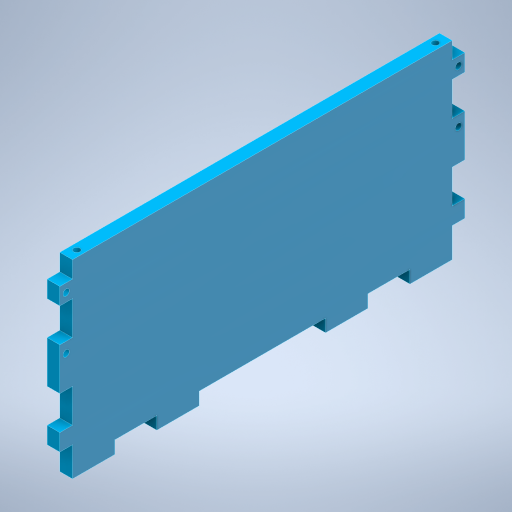
# Autodesk Inventor part: передняя стенка
Saved by Autodesk Inventor 2024.2 (Build 282272000, 272)
## iProperties
Created: 2025-11-20
Part Number: передняя стенка
Material: Типовые
Document SubType Name: Modeling
Designer: Zakhar
Density: 1 g/cm^3
Appearance: Небесно-голубой — нейтральный
Mass: 95.616 g
Surface Area: 351.84 cm^2
Volume: 95.616 cm^3
Author: Zakhar
Autodesk Inventor part; units mm, degrees
ref_plane "YZ Plane" through (0, 0, 0) normal (1, 0, 0) x (0, 1, 0)
ref_plane "XZ Plane" through (0, 0, 0) normal (0, 1, 0) x (-1, 0, 0)
ref_plane "XY Plane" through (0, 0, 0) normal (0, 0, 1) x (1, 0, 0)
sketch "Эскиз1" plane through (0, 0, 0) normal (1, 0, 0) x (0, 1, 0)
  line L0 (84, 90) -> (0, 90)
  line L1 (0, 90) -> (0, -90)
  line L2 (0, -90) -> (84, -90)
  line L3 (84, -90) -> (84, 90)
  line L4 (76, 90) -> (8, 90)
  line L5 (8, 90) -> (8, 96)
  line L6 (8, 96) -> (76, 96)
  line L7 (76, 96) -> (76, 90)
  line L8 (76, -90) -> (8, -90)
  line L9 (8, -90) -> (8, -96)
  line L10 (8, -96) -> (76, -96)
  line L11 (76, -96) -> (76, -90)
  line L12 (16, -96) -> (16, -90)
  line L13 (32, -96) -> (32, -90)
  line L14 (68, -96) -> (68, -90)
  line L15 (52, -96) -> (52, -90)
  line L16 (16, 90) -> (16, 96)
  line L17 (32, 90) -> (32, 96)
  line L18 (68, 90) -> (68, 96)
  line L19 (52, 90) -> (52, 96)
  point P0 (0, 0)
  point P1 (76, 93)
  point P2 (8, 93)
  point P3 (8, -90)
  point P4 (68, -93)
  point P5 (76, -93)
  point P6 (52, -93)
  point P7 (16, -93)
  point P8 (8, -93)
  point P9 (32, -93)
  point P10 (68, 93)
  point P11 (52, 93)
  point P12 (16, 93)
  point P13 (32, 93)
  dimension "d0" = 180
  dimension "d1" = 84
  dimension "d2" = 90
  dimension "d3" = 0
  dimension "d4" = 6
  dimension "d5" = 8
  dimension "d6" = 8
  dimension "d7" = 6
  dimension "d40" = 8
  dimension "d41" = 16
  dimension "d42" = 8
  dimension "d43" = 16
  dimension "d44" = 8
  dimension "d45" = 16
  dimension "d46" = 16
  dimension "d47" = 8
  constraints: 40 end point, 20 point on line, 12 midpoint, 11 perpendicular, 6 parallel, 3 horizontal
  measures "d0" distance of L0.end L1.end
  measures "d1" distance of L0.start L0.end
  measures "d2" distance from line of point (0, 0) L2
  measures "d3" distance from line of L1 point (0, 0)
  measures "d4" distance of L6.end L4.start
  measures "d5" horizontal distance of L0.start point (76, 93)
  measures "d6" horizontal distance of L0.end point (8, 93)
  measures "d7" distance between parallel lines of L2 L10
  measures "d40" distance of point (68, -93) point (76, -93)
  measures "d41" distance of point (52, -93) point (68, -93)
  measures "d42" distance of point (16, -93) point (8, -93)
  measures "d43" distance of point (32, -93) point (16, -93)
  measures "d44" distance of point (76, 93) point (68, 93)
  measures "d45" distance of point (52, 93) point (68, 93)
  measures "d46" distance of point (16, 93) point (32, 93)
  measures "d47" distance of point (8, 93) point (16, 93)
extrude "Выдавливание1" add sketch "Эскиз1" along normal blind 6 contours L3 L2 L1 L0 | L0 L18 L6 L7 | L11 L10 L14 L2 | L0 L17 L6 L19 | L15 L10 L13 L2 | L0 L5 L6 L16 | L12 L10 L9 L2
sketch "Эскиз4" plane through (0, 84, 90) normal (0, 1, 0) x (1, 0, 0)
  circle A0 centre (3, 5) radius 1.5
  circle A1 centre (3, 175) radius 1.5
  line L0 (0, 0) -> (6, 0)
  line L1 (6, 180) -> (6, 0)
  line L2 (0, 180) -> (6, 180)
  line L3 (6, 180) -> (6, 0) projected
  line L4 (0, 0) -> (6, 0) projected
  line L5 (0, 180) -> (6, 180) projected
  point P0 (0, 90)
  point P1 (3, 0)
  dimension "d30" = 3
  dimension "d31" = 3
  dimension "d32" = 5
  dimension "d33" = 3
  dimension "d34" = 5
  dimension "d35" = 3
  dimension "d36" = 6
  dimension "d37" = 6
  constraints: 6 end point, 3 collinear, 2 centre point, 1 midpoint
  measures "d30" diameter of A1
  measures "d31" diameter of A0
  measures "d32" distance of point (3, 0) A0.centre
  measures "d33" distance from line of L1 A0.centre
  measures "d34" distance from line of L2 A1.centre
  measures "d35" distance from line of L1 A1.centre
  measures "d36" distance of L2.start L1.start
  measures "d37" distance of L0.start L0.end
extrude "Выдавливание4" cut sketch "Эскиз4" against normal blind 4
sketch "Эскиз6" plane through (6, 0, 0) normal (1, 0, 0) x (0, 0, -1)
  line L0 (-90, 8) -> (-90, 0) projected
  line L1 (-90, 0) -> (-70, 0)
  line L2 (-70, 0) -> (-70, -6)
  line L3 (-70, -6) -> (-90, -6)
  line L4 (-90, -6) -> (-90, 0)
  line L5 (-90, 0) -> (90, 0) projected
  line L6 (-50, 0) -> (-30, 0)
  line L7 (-30, 0) -> (-30, -6)
  line L8 (-30, -6) -> (-50, -6)
  line L9 (-50, -6) -> (-50, 0)
  line L10 (30, 0) -> (50, 0)
  line L11 (50, 0) -> (50, -6)
  line L12 (50, -6) -> (30, -6)
  line L13 (30, -6) -> (30, 0)
  line L14 (90, 0) -> (70, 0)
  line L15 (70, 0) -> (70, -6)
  line L16 (70, -6) -> (90, -6)
  line L17 (90, -6) -> (90, 0)
  point P0 (0, 0)
  point P1 (-80, -6)
  point P2 (-50, -3)
  point P3 (-70, -3)
  point P4 (-30, -3)
  point P5 (90, -3)
  point P6 (70, -3)
  point P7 (50, -3)
  dimension "d48" = 6
  dimension "d49" = 6
  dimension "d50" = 6
  dimension "d51" = 20
  dimension "d52" = 20
  dimension "d53" = 20
  dimension "d54" = 20
  dimension "d55" = 20
  dimension "d56" = 20
  constraints: 32 end point, 8 parallel, 7 midpoint, 4 horizontal, 4 perpendicular, 3 point on line
  measures "d48" distance from line of L5 point (-80, -6)
  measures "d49" distance of L6.end L7.end
  measures "d50" distance of L12.end L10.start
  measures "d51" distance of L2.end L3.end
  measures "d52" distance of point (-50, -3) point (-70, -3)
  measures "d53" distance of point (-30, -3) point (-50, -3)
  measures "d54" distance of point (90, -3) point (70, -3)
  measures "d55" distance of point (70, -3) point (50, -3)
  measures "d56" distance from line of point (50, -3) L13
extrude "Выдавливание5" add sketch "Эскиз6" against normal blind 6
sketch "Эскиз7" plane through (0, 0, 0) normal (-1, 0, 0) x (0, 0, 1)
  circle A0 centre (-93, 72) radius 1.5
  line L0 (-96, 76) -> (-90, 76) projected
  line L1 (-96, 68) -> (-96, 76) projected
  circle A1 centre (-93, 47) radius 1.5
  line L2 (-96, 32) -> (-96, 52) projected
  line L3 (-96, 52) -> (-90, 52) projected
  line L4 (-96, 42) -> (96, 42) construction
  line L5 (96, 52) -> (96, 32) projected
  line L6 (-90, 84) -> (90, 84) construction
  line L7 (0, 84) -> (0, 0) construction
  circle A2 centre (93, 72) radius 1.5
  circle A3 centre (93, 47) radius 1.5
  point P0 (-96, 72)
  dimension "d59" = 4
  dimension "d60" = 3
  dimension "d61" = 3
  dimension "d62" = 3
  dimension "d63" = 3
  dimension "d64" = 5
  constraints: 4 centre point, 4 end point, 4 midpoint, 2 symmetric about line, 1 vertical, 2 other
  measures "d59" distance from line of A0.centre L0
  measures "d60" distance of point (-96, 72) A0.centre
  measures "d61" diameter of A0
  measures "d62" distance from line of L2 A1.centre
  measures "d63" diameter of A1
  measures "d64" distance from line of L3 A1.centre
extrude "Выдавливание6" cut sketch "Эскиз7" against normal blind 6
equation "\"d2\" = 0.5 * d0"
equation "\"d42\" = d40"
equation "\"d43\" = d41"
equation "\"d44\" = d40"
equation "\"d45\" = d41"
equation "\"d46\" = d41"
equation "\"d47\" = d40"
equation "\"d52\" = d51"
equation "\"d53\" = d51"
equation "\"d54\" = d51"
equation "\"d55\" = d51"
equation "\"d56\" = d51"
